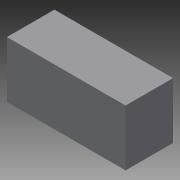
# Autodesk Inventor part: gear_lock
Saved by Autodesk Inventor 2013 (Build 170138000, 138)
## iProperties
Created: 2015-09-10
Part Number: gear_lock
Material: Generic
Document SubType Name: Modeling
Designer: Students
Density: 1 g/cm^3
Author: Students
Autodesk Inventor part; units mm, degrees
ref_plane "YZ Plane" through (0, 0, 0) normal (1, 0, 0) x (0, 1, 0)
ref_plane "XZ Plane" through (0, 0, 0) normal (0, 1, 0) x (-1, 0, 0)
ref_plane "XY Plane" through (0, 0, 0) normal (0, 0, 1) x (1, 0, 0)
sketch "Sketch1" plane through (0, 0, 0) normal (0, 1, 0) x (-1, 0, 0)
  line L0 (0, 0) -> (-15, 0)
  line L1 (-15, 0) -> (-15, -7.1)
  line L2 (-15, -7.1) -> (0, -7.1)
  line L3 (0, -7.1) -> (0, 0)
  dimension "d0" = 15
  dimension "d1" = 7.1
  constraints: 8 end point, 2 parallel, 1 horizontal, 1 perpendicular
  measures "d0" distance of L2.end L1.end
  measures "d1" distance of L1.end L0.end
extrude "Extrusion1" add sketch "Sketch1" along normal blind 6
body "Solid1"
